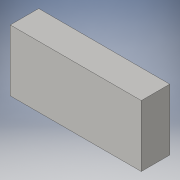
# Autodesk Inventor part: mcdave battery
Saved by Autodesk Inventor 2016 (Build 200138000, 138)
## iProperties
Created: 2016-10-05
Part Number: mcdave battery
Material: Generic
Document SubType Name: Modeling
Designer: ClenoR
Density: 1 g/cm^3
Appearance: Default
Author: ClenoR
Autodesk Inventor part; units mm, degrees
ref_plane "YZ Plane" through (0, 0, 0) normal (1, 0, 0) x (0, 1, 0)
ref_plane "XZ Plane" through (0, 0, 0) normal (0, 1, 0) x (-1, 0, 0)
ref_plane "XY Plane" through (0, 0, 0) normal (0, 0, 1) x (1, 0, 0)
sketch "Sketch1" plane through (0, 0, 0) normal (0, 0, 1) x (1, 0, 0)
  line L0 (-39.5395, 13.5006) -> (30.4629, 13.5006)
  line L1 (30.4629, 13.5006) -> (30.4629, -19.3162)
  line L2 (30.4629, -19.3162) -> (-39.5395, -19.3162)
  line L3 (-39.5395, -19.3162) -> (-39.5395, 13.5006)
  point P0 (0, 0)
  dimension "d0" = 32.8168
  dimension "d1" = 70.0024
  constraints: 8 end point, 2 parallel, 1 horizontal, 1 perpendicular
  measures "d0" distance of L0.end L1.end
  measures "d1" distance of L0.start L0.end
extrude "Extrusion1" add sketch "Sketch1" along normal blind 15.1892
body "Solid1"
